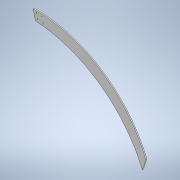
# Autodesk Inventor part: spoke2
Saved by Autodesk Inventor 2020.3 (Build 243373000, 373)
## iProperties
Created: 2020-11-01
Part Number: spoke2
Material: Generic
Document SubType Name: Modeling
Designer: Martijn
Density: 1 g/cm^3
Appearance: Default
Mass: 78.3877 g
Surface Area: 437.313 cm^2
Volume: 78.3877 cm^3
Author: Martijn
Autodesk Inventor part; units mm, degrees
ref_plane "YZ Plane" through (0, 0, 0) normal (1, 0, 0) x (0, 1, 0)
ref_plane "XZ Plane" through (0, 0, 0) normal (0, 1, 0) x (-1, 0, 0)
ref_plane "XY Plane" through (0, 0, 0) normal (0, 0, 1) x (1, 0, 0)
sketch "Sketch1" plane through (0, 0, 0) normal (0, 0, 1) x (1, 0, 0)
  arc A0 (670.9948, -199.4141) -> (0, 0) centre (254.9219, -370.8299) ccw
  arc A1 (657.7848, -239.4141) -> (30, 0) centre (229.3296, -420.1103) ccw
  arc A2 (657.7848, -239.4141) -> (670.9948, -199.4141) centre (0, 0) ccw
  line L0 (0, 0) -> (30, 0)
  line L1 (657.7848, -239.4141) -> (0, 0)
  line L2 (-143.7228, 0) -> (862.3369, 0) projected
  point P0 (0, 0)
  dimension "d1" = 30
  dimension "d2" = 40
  dimension "d4" = 20
  dimension "d5" = 465
  dimension "d6" = 450
  dimension "d22" = 700
  constraints: 6 point on circle, 4 end point, 3 centre point, 1 coincident, 1 horizontal
  measures "d1" distance of L0.start L0.end
  measures "d2" vertical distance of L1.start A0.start
  measures "d4" angle of L1 L2
  measures "d5" radius of A1
  measures "d6" radius of A0
  measures "d22" radius of A2
extrude "Extrusion1" add sketch "Sketch1" along normal blind 4 contours A2 A1 L2 A0 | L2 A1 L0 A0
sketch "Sketch2" plane through (0, 0, 4) normal (0, 0, 1) x (1, 0, 0)
  arc A0 (670.9948, -199.4141) -> (0, 0) centre (254.9219, -370.8299) ccw projected
  arc A1 (87.1309, 22.5434) -> (74.166, 50.9844) centre (0, 0) ccw
  line L0 (74.166, 50.9844) -> (0, 0)
  line L1 (0, 0) -> (87.1309, 22.5434)
  line L2 (0, 0) -> (30, 0) projected
  point P0 (78.8927, 43.3122)
  point P1 (0, 0)
  point P2 (0, 0)
  dimension "d9" = 90
  dimension "d16" = 20
  constraints: 4 end point, 2 point on circle, 1 centre point, 1 coincident, 1 tangent
  measures "d9" distance of L2.start L1.end
  measures "d16" angle of L1 L0
extrude "Extrusion2" add sketch "Sketch2" against normal blind 4
sketch "Sketch4" plane through (0, 0, 4) normal (0, 0, 1) x (1, 0, 0)
  line L0 (86.0304, 22.2587) -> (87.1309, 22.5434) projected
  line L1 (74.166, 50.9844) -> (0, 0) projected
  line L2 (87.1309, 22.5434) -> (0, 0)
  line L3 (0, 0) -> (30, 0)
  arc A0 (86.0304, 22.2587) -> (30, 0) centre (229.3296, -420.1103) ccw projected
  line L4 (30, 0) -> (86.0304, 22.2587)
  point P0 (86.0304, 22.2587)
  constraints: 6 end point, 1 horizontal
extrude "Extrusion4" cut sketch "Sketch4" against normal blind 10 contours A0 L3 L2
sketch "Sketch5" plane through (0, 0, 4) normal (0, 0, 1) x (1, 0, 0)
  line L0 (0, 0) -> (8.2407, 5.6649)
  line L1 (74.166, 50.9844) -> (0, 0) projected
  line L2 (0, 0) -> (87.1309, 22.5434) projected
  line L3 (9.6812, 2.5048) -> (0, 0)
  arc A0 (9.6812, 2.5048) -> (8.2407, 5.6649) centre (0, 0) ccw
  point P0 (9.6812, 2.5048)
  dimension "d21" = 10
  constraints: 4 end point, 2 coincident, 2 point on circle, 1 centre point, 1 collinear, 1 point on line
  measures "d21" radius of A0
extrude "Extrusion5" cut sketch "Sketch5" against normal blind 10
sketch "Sketch6" plane through (0, 0, 4) normal (0, 0, 1) x (1, 0, 0)
  arc A0 (670.9948, -199.4141) -> (78.8927, 43.3122) centre (254.9219, -370.8299) ccw projected
  arc A1 (258.8056, -24.8926) -> (214.2573, 147.2882) centre (0, 0) ccw
  line L0 (0, 0) -> (214.2573, 147.2882)
  line L1 (0, 0) -> (258.8056, -24.8926)
  line L2 (74.166, 50.9844) -> (8.2407, 5.6649) projected
  dimension "d23" = 40
  dimension "d24" = 260
  constraints: 4 end point, 2 point on circle, 1 centre point, 1 coincident, 1 collinear
  measures "d23" angle of L1 L0
  measures "d24" radius of A1
extrude "Extrusion6" cut sketch "Sketch6" against normal blind 10
sketch "Sketch7" plane through (0, 0, 4) normal (0, 0, 1) x (1, 0, 0)
  line L0 (0, 0) -> (260.1676, 72.1998)
  line L1 (0, 0) -> (264.5703, 53.8755)
  line L2 (-134.199, 0) -> (805.1938, 0) projected
  circle A0 centre (260.1676, 72.1998) radius 1.5
  circle A1 centre (264.5703, 53.8755) radius 1.5
  circle A2 centre (281.223, 70.1761) radius 1.5
  circle A3 centre (285.6257, 51.8518) radius 1.5
  line L3 (281.223, 70.1761) -> (285.6257, 51.8518)
  line L4 (285.6257, 51.8518) -> (264.5703, 53.8755)
  line L5 (264.5703, 53.8755) -> (260.1676, 72.1998)
  line L6 (281.223, 70.1761) -> (260.1676, 72.1998)
  dimension "d27" = 15.51
  dimension "d28" = 4
  dimension "d29" = 270
  dimension "d30" = 270
  dimension "d31" = 3
  dimension "d32" = 3
  dimension "d33" = 3
  dimension "d34" = 3
  dimension "d35" = 109
  dimension "d36" = 20
  constraints: 12 end point, 4 centre point, 2 parallel, 1 coincident
  measures "d27" angle of L2 L0
  measures "d28" angle of L0 L1
  measures "d29" distance of L0.start L1.end
  measures "d30" distance of L0.start L0.end
  measures "d31" diameter of A0
  measures "d32" diameter of A1
  measures "d33" diameter of A2
  measures "d34" diameter of A3
  measures "d35" angle of L5 L4
  measures "d36" distance between parallel lines of L5 L3
extrude "Extrusion7" cut sketch "Sketch7" against normal through all contours A0 L6 L0 | L0 L5 A0 | A1 L5 L1 | L1 L4 A1 | L6 A0 L5 | L5 A1 L4 | L4 L3 A3 | A3 L3 L4 | L6 L3 A2 | A2 L3 L6
body "Solid1"
